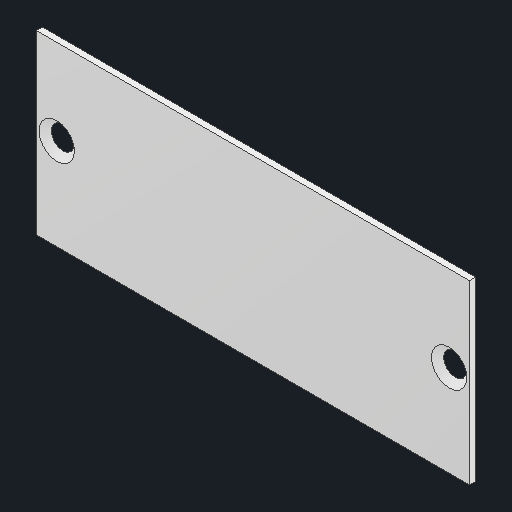
# Autodesk Inventor part: back
Saved by Autodesk Inventor 2023 (Build 270158000, 158)
## iProperties
Created: 2024-05-26
Part Number: back
Material: ABS Plastic
Document SubType Name: Modeling
Designer: szymo
Density: 1.06 g/cm^3
Appearance: Smooth - White
Mass: 2.14362 g
Surface Area: 42.8513 cm^2
Volume: 2.02229 cm^3
Author: szymo
Autodesk Inventor part; units mm, degrees
ref_plane "YZ Plane" through (0, 0, 0) normal (1, 0, 0) x (0, 1, 0)
ref_plane "XZ Plane" through (0, 0, 0) normal (0, 1, 0) x (-1, 0, 0)
ref_plane "XY Plane" through (0, 0, 0) normal (0, 0, 1) x (1, 0, 0)
sketch "Sketch1" plane through (0, 0, 0) normal (0, 0, 1) x (1, 0, 0)
  line L0 (-28.5, 29) -> (42.5, 29)
  line L1 (42.5, 29.0093) -> (42.5, 0)
  line L2 (42.5, 0) -> (-28.5, 0)
  line L3 (-28.5, 0) -> (-28.5, 29)
  circle A0 centre (-25.15, 15) radius 1.75 projected
  line L4 (-28.5, 29) -> (-21.8, 29) projected
  line L5 (-28.5, 29) -> (-28.5, 25.5) projected
  line L6 (-28.5, 25.5) -> (-28.5, 0) projected
  line L7 (-28.5, 0) -> (-21.8, 0) projected
  line L8 (-21.8, 0) -> (-21.8, 29) projected
  circle A1 centre (39.15, 15) radius 1.75 projected
  line L9 (42.5, 29) -> (35.8, 29) projected
  line L10 (35.8, 0) -> (35.8, 29) projected
  line L11 (42.5, 0) -> (35.8, 0) projected
  line L12 (42.5, 25.5) -> (42.5, 0) projected
  line L13 (42.5, 29) -> (42.5, 25.5) projected
  point P0 (0, 0)
  point P1 (-22.8, 0)
  constraints: 8 end point, 5 collinear, 2 parallel, 1 horizontal, 1 perpendicular, 1 point on line
extrude "Extrusion1" add sketch "Sketch1" along normal blind 1 contours L0 L8 L2 L3 | L0 L10 L2 L8 | L0 L1 L2 L10 | A0 | A1
sketch "Sketch2" plane through (0, 0, 1) normal (0, 0, 1) x (1, 0, 0)
  circle A0 centre (-25.15, 15) radius 1.75 projected
  circle A1 centre (39.15, 15) radius 1.75 projected
  point P0 (0, 0)
  constraints: 2 coincident
hole "Hole1" at (-25.15, 15, 1) at (39.15, 15, 1) direction (0, 0, -1) diameter 3.1 end through all countersink diameter 5.8 countersink angle 90 clearance for "Countersunk Flat Head Screw ISO 2009/7046" size "M2.5" standard "ISO"
body "Solid1"
